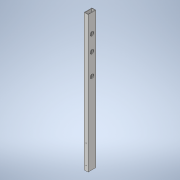
# Autodesk Inventor part: 16in 2x1 Aluminum Block-ver1-1111-2019
Saved by Autodesk Inventor 2021 (Build 250183000, 183)
## iProperties
Created: 2020-01-17
Part Number: 16in 2x1 Aluminum Block-ver1-1111-2019
Material: Generic
Document SubType Name: Modeling
Designer: JMHal
Density: 1 g/cm^3
Appearance: Default
Author: JMHal
Autodesk Inventor part; units mm, degrees
ref_plane "YZ Plane" through (0, 0, 0) normal (1, 0, 0) x (0, 1, 0)
ref_plane "XZ Plane" through (0, 0, 0) normal (0, 1, 0) x (-1, 0, 0)
ref_plane "XY Plane" through (0, 0, 0) normal (0, 0, 1) x (1, 0, 0)
sketch "Sketch1" plane through (0, 0, 0) normal (0, 1, 0) x (-1, 0, 0)
  line L0 (0, 0) -> (25.4, 0)
  line L1 (25.4, 0) -> (25.4, -50.8)
  line L2 (25.4, -50.8) -> (0, -50.8)
  line L3 (0, -50.8) -> (0, 0)
  line L4 (3.175, -3.175) -> (22.225, -3.175)
  line L5 (22.225, -3.175) -> (22.225, -47.625)
  line L6 (22.225, -47.625) -> (3.175, -47.625)
  line L7 (3.175, -47.625) -> (3.175, -3.175)
  dimension "d0" = 50.8
  dimension "d1" = 25.4
  dimension "d2" = 3.175
  constraints: 16 end point, 4 parallel, 2 perpendicular, 1 horizontal, 3 other
  measures "d0" distance between parallel lines of L2 L0
  measures "d1" distance between parallel lines of L3 L1
  measures "d2" distance between parallel lines of L3 L7
extrude "Extrusion1" add sketch "Sketch1" along normal blind 889
sketch "Sketch6" plane through (0, 0, 0) normal (1, 0, 0) x (0, 0, -1)
  circle A0 centre (25.4, 768.35) radius 12.7
  line L0 (0, 889) -> (50.8, 889) projected
  line L1 (0, 0) -> (0, 889) projected
  dimension "d5" = 25.4
  dimension "d6" = 120.65
  dimension "d7" = 25.4
  constraints: 1 centre point
  measures "d5" diameter of A0
  measures "d6" distance from line of A0.centre L0
  measures "d7" distance from line of L1 A0.centre
extrude "Extrusion2" cut sketch "Sketch6" against normal blind 25.4
sketch "Sketch8" plane through (-25.4, 0, 0) normal (0, 0, 1) x (1, 0, 0)
  circle A0 centre (12.7, 31.75) radius 2.0701
  line L0 (0, 0) -> (0, 889) projected
  line L1 (25.4, 0) -> (0, 0) projected
  dimension "d13" = 4.1402
  dimension "d14" = 12.7
  dimension "d15" = 31.75
  constraints: 1 centre point
  measures "d13" diameter of A0
  measures "d14" distance from line of A0.centre L0
  measures "d15" distance from line of L1 A0.centre
extrude "Extrusion3" cut sketch "Sketch8" against normal blind 76.2
sketch "Sketch9" plane through (-25.4, 0, 0) normal (0, 0, 1) x (1, 0, 0)
  circle A0 centre (12.7, 157.5054) radius 2.0701
  line L0 (25.4, 0) -> (0, 0) projected
  line L1 (0, 0) -> (0, 889) projected
  dimension "d18" = 4.1402
  dimension "d19" = 157.5054
  dimension "d20" = 12.7
  constraints: 1 centre point
  measures "d18" diameter of A0
  measures "d19" distance from line of L0 A0.centre
  measures "d20" distance from line of A0.centre L1
extrude "Extrusion4" cut sketch "Sketch9" against normal blind 76.2
sketch "Sketch10" plane through (0, 0, 0) normal (1, 0, 0) x (0, 0, -1)
  circle A0 centre (25.4, 528.066) radius 12.7
  line L0 (50.8, 0) -> (50.8, 889) projected
  line L1 (50.8, 0) -> (0, 0) projected
  circle A1 centre (25.4, 666.75) radius 12.7
  dimension "d23" = 25.4
  dimension "d24" = 25.4
  dimension "d25" = 528.066
  dimension "d26" = 25.4
  dimension "d27" = 666.75
  constraints: 2 centre point
  measures "d23" diameter of A0
  measures "d24" distance from line of L0 A0.centre
  measures "d25" distance from line of L1 A0.centre
  measures "d26" diameter of A1
  measures "d27" distance from line of L1 A1.centre
extrude "Extrusion5" cut sketch "Sketch10" against normal blind 25.4
body "Solid1"
